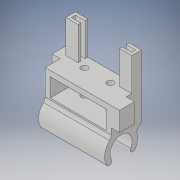
# Autodesk Inventor part: Roller_Switch._new
Saved by Autodesk Inventor 2019 (Build 230136000, 136)
## iProperties
Created: 2019-10-10
Part Number: Roller_Switch._new
Material: Generic
Document SubType Name: Modeling
Designer: James
Density: 1 g/cm^3
Appearance: Default
Author: James
Autodesk Inventor part; units mm, degrees
ref_plane "YZ Plane" through (0, 0, 0) normal (1, 0, 0) x (0, 1, 0)
ref_plane "XZ Plane" through (0, 0, 0) normal (0, 1, 0) x (-1, 0, 0)
ref_plane "XY Plane" through (0, 0, 0) normal (0, 0, 1) x (1, 0, 0)
sketch "Sketch1" plane through (0, 0, 0) normal (1, 0, 0) x (0, 1, 0)
  circle A0 centre (0, 0) radius 4
  arc A1 (-3, -5.1962) -> (-3, 5.1962) centre (0, 0) ccw
  arc A2 (-3, 5.1962) -> (-2, 3.4641) centre (-2.5, 4.3301) ccw
  arc A3 (-2, -3.4641) -> (-3, -5.1962) centre (-2.5, -4.3301) ccw
  line L0 (15, 3.6) -> (4, 3.6)
  line L1 (4, 3.6) -> (4, -7.4)
  line L2 (4, -7.4) -> (15, -7.4)
  line L3 (15, -7.4) -> (15, 3.6)
  dimension "d0" = 8
  dimension "d1" = 12
  dimension "d2" = 2.5
  dimension "d4" = 11
  dimension "d5" = 11
  dimension "d6" = 4
  dimension "d9" = 7.4
  constraints: 8 end point, 8 point on circle, 4 centre point, 4 tangent, 2 coincident, 2 parallel, 1 horizontal, 1 perpendicular, 1 vertical alignment
  measures "d0" diameter of A0
  measures "d1" diameter of A1
  measures "d2" horizontal distance of A3.centre point (0, 0)
  measures "d4" distance of L2.end L0.start
  measures "d5" distance of L0.start L0.end
  measures "d6" distance from line of point (0, 0) L1
  measures "d9" distance from line of point (0, 0) L2
extrude "Extrusion1" add sketch "Sketch1" along normal blind 24 contours L1 A1 A3 A0 | A0 A2 A1 L0 L1 | L1 L0 A1 | A1 L0 L3 L2 L1
sketch "Sketch2" plane through (0, 4.8, 3.6) normal (0, 0, 1) x (1, 0, 0)
  line L0 (1.8, 8.2) -> (22.2, 8.2)
  line L1 (22.2, 8.2) -> (22.2, 1.5)
  line L2 (22.2, 1.5) -> (1.8, 1.5)
  line L3 (1.8, 1.5) -> (1.8, 8.2)
  line L4 (0, 10.2) -> (24, 10.2) projected
  point P0 (0, -4.8)
  point P1 (12, 8.2)
  point P2 (12, 10.2)
  dimension "d10" = 20.4
  dimension "d11" = 6.7
  dimension "d12" = 13
  constraints: 8 end point, 2 midpoint, 2 parallel, 1 horizontal, 1 perpendicular, 1 vertical alignment
  measures "d10" distance of L0.start L0.end
  measures "d11" distance of L2.end L0.start
  measures "d12" distance from line of point (0, -4.8) L0
extrude "Extrusion2" cut sketch "Sketch2" against normal blind 10
fillet "Fillet1" radius 2 1 edges at (12, 4, -4.4721)
fillet "Fillet2" radius 2 1 edges at (12, 4.8, 3.6)
sketch "Sketch3" plane through (0, 4.8, -6.4) normal (0, 0, 1) x (1, 0, 0)
  line L0 (1.8, 8.2) -> (22.2, 8.2) projected
  line L1 (22.2, 0.9418) -> (1.8, 0.9418) projected
  line L2 (2.2, 8.2) -> (5.4, 8.2)
  line L3 (5.4, 8.2) -> (5.4, 0.9418)
  line L4 (5.4, 0.9418) -> (2.2, 0.9418)
  line L5 (2.2, 0.9418) -> (2.2, 8.2)
  line L6 (11, 8.2) -> (14.2, 8.2)
  line L7 (14.2, 8.2) -> (14.2, 0.9418)
  line L8 (14.2, 0.9418) -> (11, 0.9418)
  line L9 (11, 0.9418) -> (11, 8.2)
  line L10 (18.3, 8.2) -> (21.5, 8.2)
  line L11 (21.5, 8.2) -> (21.5, 0.9418)
  line L12 (21.5, 0.9418) -> (18.3, 0.9418)
  line L13 (18.3, 0.9418) -> (18.3, 8.2)
  line L14 (1.8, 1.5) -> (1.8, 8.2) projected
  point P0 (0, -4.8)
  point P1 (3.8, 8.2)
  point P2 (12.6, 8.2)
  point P3 (19.9, 8.2)
  point P4 (1.8, 1.1156)
  dimension "d17" = 3.2
  dimension "d18" = 3.2
  dimension "d19" = 3.2
  dimension "d20" = 2
  dimension "d21" = 8.8
  dimension "d22" = 7.3
  constraints: 24 end point, 6 parallel, 6 point on line, 3 horizontal, 3 midpoint, 3 perpendicular
  measures "d17" distance between parallel lines of L3 L5
  measures "d18" distance between parallel lines of L7 L9
  measures "d19" distance between parallel lines of L11 L13
  measures "d20" distance from line of point (3.8, 8.2) L14
  measures "d21" distance of point (12.6, 8.2) point (3.8, 8.2)
  measures "d22" distance of point (19.9, 8.2) point (12.6, 8.2)
extrude "Extrusion3" cut sketch "Sketch3" against normal blind 10 contours L0 L3 L1 L5 | L0 L7 L1 L9 | L0 L11 L1 L13
sketch "Sketch4" plane through (0, 15, 3.6) normal (0, 1, 0) x (1, 0, 0)
  circle A0 centre (7.25, 7) radius 1.2
  circle A1 centre (16.75, 7) radius 1.2
  line L0 (0, 11) -> (24, 11) projected
  point P0 (0, 3.6)
  point P1 (12, 11)
  dimension "d25" = 2.4
  dimension "d26" = 9.5
  dimension "d27" = 4.75
  dimension "d28" = 4
  constraints: 2 centre point, 1 equal radius, 1 horizontal alignment, 1 midpoint
  measures "d25" diameter of A0
  measures "d26" distance of A1.centre A0.centre
  measures "d27" horizontal distance of point (12, 11) A0.centre
  measures "d28" distance from line of A0.centre L0
extrude "Extrusion4" cut sketch "Sketch4" against normal blind 10.5
sketch "Sketch5" plane through (24, 0, 0) normal (1, 0, 0) x (0, 0, -1)
  line L0 (-3.6, 15) -> (-3.6, 5.7131) projected
  line L1 (-3.6, 15) -> (1.9, 15)
  line L2 (1.9, 15) -> (1.9, 8)
  line L3 (1.9, 8) -> (-3.6, 8)
  line L4 (-3.6, 8) -> (-3.6, 15)
  point P0 (0, 0)
  dimension "d31" = 5.5
  dimension "d32" = 7
  constraints: 8 end point, 2 parallel, 1 horizontal, 1 perpendicular
  measures "d31" distance of L0.start L1.end
  measures "d32" distance of L1.end L2.end
extrude "Extrusion5" add sketch "Sketch5" along normal blind 3
sketch "Sketch6" plane through (0, 0, 0) normal (-1, 0, 0) x (0, 0, 1)
  line L0 (-7.4, 4) -> (-7.4, 15) projected
  line L1 (-7.4, 15) -> (-1.9, 15)
  line L2 (-1.9, 15) -> (-1.9, 8)
  line L3 (-1.9, 8) -> (-7.4, 8)
  line L4 (-7.4, 8) -> (-7.4, 15)
  point P0 (0, 0)
  point P1 (-8, 4)
  dimension "d35" = 7
  dimension "d36" = 5.5
  constraints: 8 end point, 2 parallel, 1 horizontal, 1 perpendicular, 1 other
  measures "d35" distance of L1.end L2.end
  measures "d36" distance of L2.end L3.end
extrude "Extrusion6" add sketch "Sketch6" along normal blind 3
sketch "Sketch11" plane through (0, 15, 3.6) normal (0, 1, 0) x (1, 0, 0)
  line L0 (0, 11) -> (24, 11) projected
  line L1 (0, 5.5) -> (0, 11) projected
  line L2 (0, 11) -> (0, 7.5)
  line L3 (24, 7.5) -> (24, 11)
  line L4 (1, 8.5) -> (1, 10)
  line L5 (23, 10) -> (23, 8.5)
  line L6 (19.5, 8.5) -> (19.5, 7.5)
  line L7 (19.5, 10) -> (19.5, 11)
  line L8 (-3, 11) -> (24, 11) projected
  line L9 (4.5, 7.5) -> (4.5, 8.5)
  line L10 (4.5, 10) -> (4.5, 11)
  line L11 (19.5, 10) -> (19.5, 11)
  line L12 (18.3, 11) -> (21.5, 11) projected
  line L13 (1, 10) -> (4.5, 10)
  line L14 (19.5, 10) -> (23, 10)
  line L15 (24, 11) -> (19.5, 11)
  line L16 (4.5, 11) -> (0, 11)
  line L17 (23, 8.5) -> (19.5, 8.5)
  line L18 (4.5, 8.5) -> (1, 8.5)
  line L19 (0, 7.5) -> (4.5, 7.5)
  line L20 (19.5, 7.5) -> (24, 7.5)
  point P0 (0, 3.6)
  point P1 (23, 9.25)
  point P2 (24, 9.4038)
  point P3 (24, 9.25)
  point P4 (1, 9.25)
  point P5 (21.75, 7.5)
  point P6 (2.25, 7.5)
  point P7 (2.75, 8.5)
  point P8 (21.25, 8.5)
  point P9 (21.25, 10)
  point P10 (2.75, 10)
  point P11 (21.75, 11)
  point P12 (2.25, 11)
  dimension "d62" = 1.5
  dimension "d63" = 1
  dimension "d64" = 15
  dimension "d70" = 4.5
  dimension "d71" = 3.5
  dimension "d72" = 1
  constraints: 34 end point, 11 midpoint, 10 parallel, 9 perpendicular, 6 horizontal alignment, 6 point on line, 4 horizontal
  measures "d62" distance of L5.start L5.end
  measures "d63" distance between parallel lines of L3 L5
  measures "d64" distance between parallel lines of L9 L6
  measures "d70" distance between parallel lines of L6 L3
  measures "d71" distance of L3.start L0.end
  measures "d72" distance between parallel lines of L1 L4
extrude "Extrusion10" add sketch "Sketch11" along normal blind 12
body "Solid1"
